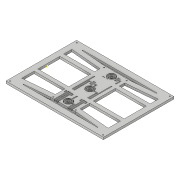
# Autodesk Inventor part: LD_holder_p11
Saved by Autodesk Inventor 2022 (Build 260153000, 153)
## iProperties
Created: 2020-08-30
Part Number: LD_holder_p11
Material: Generic
Document SubType Name: Modeling
Designer: LIU
Density: 1 g/cm^3
Appearance: Default
Author: LIU
Autodesk Inventor part; units mm, degrees
ref_plane "YZ Plane" through (0, 0, 0) normal (1, 0, 0) x (0, 1, 0)
ref_plane "XZ Plane" through (0, 0, 0) normal (0, 1, 0) x (-1, 0, 0)
ref_plane "XY Plane" through (0, 0, 0) normal (0, 0, 1) x (1, 0, 0)
sketch "Sketch1" plane through (0, 0, 0) normal (0, 1, 0) x (-1, 0, 0)
  line L0 (0, -89.88) -> (0, 89.88) construction
  line L1 (124.04, 0) -> (-124.04, 0) construction
  line L2 (0, 15.386221) -> (0, -13.818145) construction
  circle A0 centre (0, 0) radius 1.85
  circle A1 centre (0, -39.2) radius 1.85
  circle A2 centre (0, 39.2) radius 1.85
  line L3 (-22.5, 49.2) -> (22.5, 49.2)
  line L4 (22.5, 49.2) -> (22.5, 40.666307) construction
  line L5 (22.5, -49.2) -> (-22.5, -49.2)
  line L6 (-22.5, -49.2) -> (-22.5, -40.666307) construction
  line L7 (-22.5, 49.2) -> (22.5, -49.2) construction
  line L8 (22.5, 49.2) -> (-22.5, -49.2) construction
  line L9 (-78.6, 54.2) -> (78.6, 54.2)
  line L10 (78.6, 54.2) -> (78.6, 45.666307) construction
  line L11 (78.6, -54.2) -> (-78.6, -54.2)
  line L12 (-78.6, -54.2) -> (-78.6, -45.666307) construction
  line L13 (-78.6, 54.2) -> (78.6, -54.2) construction
  line L14 (78.6, 54.2) -> (-78.6, -54.2) construction
  line L15 (-88.6, 64.2) -> (88.6, 64.2)
  line L16 (88.6, 64.2) -> (88.6, -64.2)
  line L17 (88.6, -64.2) -> (-88.6, -64.2)
  line L18 (-88.6, -64.2) -> (-88.6, 64.2)
  line L19 (-88.6, 64.2) -> (88.6, -64.2) construction
  line L20 (88.6, 64.2) -> (-88.6, -64.2) construction
  line L21 (22.5, -49.2) -> (78.6, -54.2)
  line L22 (22.5, -40.666307) -> (78.6, -45.666307)
  line L23 (22.5, 49.2) -> (78.6, 54.2)
  line L24 (22.5, 40.666307) -> (78.6, 45.666307)
  line L25 (-22.5, -49.2) -> (-78.6, -54.2)
  line L26 (-22.5, -40.666307) -> (-78.6, -45.666307)
  line L27 (-22.5, 40.666307) -> (-78.6, 45.666307)
  line L28 (-22.5, 49.2) -> (-78.6, 54.2)
  circle A3 centre (20.5, 46.2) radius 1
  circle A4 centre (20.5, -46.2) radius 1
  circle A5 centre (-20.5, 46.2) radius 1
  circle A6 centre (-20.5, -46.2) radius 1
  line L29 (78.6, 45.666307) -> (78.6, -45.666307)
  line L30 (78.6, -45.666307) -> (78.6, -54.2) construction
  line L31 (22.5, 40.666307) -> (22.5, -40.666307)
  line L32 (22.5, -40.666307) -> (22.5, -49.2) construction
  line L33 (-22.5, 40.666307) -> (-22.5, 49.2) construction
  line L34 (-22.5, -40.666307) -> (-22.5, 40.666307)
  line L35 (-78.6, 45.666307) -> (-78.6, 54.2) construction
  line L36 (-78.6, -45.666307) -> (-78.6, 45.666307)
  dimension "d0" = 0
  dimension "d1" = 3.7
  dimension "d2" = 3.7
  dimension "d3" = 3.7
  dimension "d4" = 39.2
  dimension "d5" = 39.2
  dimension "d6" = 45
  dimension "d7" = 98.4
  dimension "d8" = 5
  dimension "d9" = 56.1
  dimension "d10" = 10
  dimension "d11" = 10
  dimension "d12" = 8.5
  dimension "d13" = 2
  dimension "d14" = 2
  dimension "d15" = 3
  constraints: 70 end point, 23 parallel, 9 symmetric about line, 7 centre point, 7 midpoint, 7 perpendicular, 5 point on line, 3 horizontal, 1 collinear, 3 other
  measures "d0" distance between parallel lines of L0 L2
  measures "d1" diameter of A0
  measures "d2" diameter of A1
  measures "d3" diameter of A2
  measures "d4" distance of A0.centre A1.centre
  measures "d5" distance of A0.centre A2.centre
  measures "d6" distance of L5.start L5.end
  measures "d7" distance of L3.end L5.start
  measures "d8" distance between parallel lines of L11 L5
  measures "d9" distance between parallel lines of L4 L10
  measures "d10" distance between parallel lines of L16 L10
  measures "d11" distance between parallel lines of L11 L17
  measures "d12" distance between parallel lines of L21 L22
  measures "d13" distance from line of L4 A3.centre
  measures "d14" diameter of A3
  measures "d15" distance from line of L3 A3.centre
extrude "Extrusion1" add sketch "Sketch1" along normal blind 4
fillet "Fillet1" radius 0.5 4 edges at (78.6, 2, 54.2) (-78.6, 2, 54.2) (-78.6, 2, -54.2) (78.6, 2, -54.2)
sketch "Sketch2" plane through (0, 4, 0) normal (0, 1, 0) x (1, 0, 0)
  circle A0 centre (0, -39.2) radius 1.85 projected
  circle A1 centre (0, 39.2) radius 1.85 projected
  circle A2 centre (0, 0) radius 1.85 projected
  circle A3 centre (0, -39.2) radius 2.9
  circle A4 centre (0, 0) radius 2.9
  circle A5 centre (0, 39.2) radius 2.9
  dimension "d19" = 5.8
  dimension "d20" = 5.8
  dimension "d21" = 5.8
  constraints: 3 centre point, 3 coincident
  measures "d19" diameter of A3
  measures "d20" diameter of A4
  measures "d21" diameter of A5
extrude "Extrusion2" cut sketch "Sketch2" against normal blind 1.6
sketch "Sketch3" plane through (0, 4, 0) normal (0, 1, 0) x (1, 0, 0)
  line L0 (-88.6, -64.2) -> (88.6, -64.2) projected
  line L1 (-88.6, 64.2) -> (-88.6, -64.2) projected
  circle A0 centre (-84.6, -60.7) radius 1
  line L2 (0, 89.88) -> (0, -89.88) projected
  line L3 (-124.04, 0) -> (124.04, 0) projected
  circle A1 centre (-84.6, 60.7) radius 1
  circle A2 centre (84.6, -60.7) radius 1
  circle A3 centre (84.6, 60.7) radius 1
  point P0 (0, 0)
  dimension "d24" = 4
  dimension "d25" = 3.5
  dimension "d26" = 2
  constraints: 4 centre point, 3 symmetric about line, 3 other
  measures "d24" distance from line of L1 A0.centre
  measures "d25" distance from line of L0 A0.centre
  measures "d26" diameter of A0
extrude "Extrusion3" cut sketch "Sketch3" against normal through all contours A0 | A1 | A2 | A3
sketch "Sketch4" plane through (0, 0, 0) normal (0, -1, 0) x (1, 0, 0)
  circle A0 centre (84.6, 60.7) radius 1
  circle A1 centre (-84.6, 60.7) radius 1
  circle A2 centre (-84.6, -60.7) radius 1
  circle A3 centre (84.6, -60.7) radius 1
  line L0 (-88.6, 64.2) -> (-88.6, -64.2)
  line L1 (-84.6, -58.332864) -> (-82.55, -59.516432)
  line L2 (-82.55, -59.516432) -> (-82.55, -61.883568)
  line L3 (-82.55, -61.883568) -> (-84.6, -63.067136)
  line L4 (-84.6, -63.067136) -> (-86.65, -61.883568)
  line L5 (-86.65, -61.883568) -> (-86.65, -59.516432)
  line L6 (-86.65, -59.516432) -> (-84.6, -58.332864)
  line L7 (0, -89.88) -> (0, 89.88)
  line L8 (-124.04, 0) -> (124.04, 0)
  circle A4 centre (-84.6, 60.7) radius 1
  line L9 (-84.6, 58.332864) -> (-82.55, 59.516432)
  line L10 (-82.55, 59.516432) -> (-82.55, 61.883568)
  line L11 (-82.55, 61.883568) -> (-84.6, 63.067136)
  line L12 (-84.6, 63.067136) -> (-86.65, 61.883568)
  line L13 (-86.65, 61.883568) -> (-86.65, 59.516432)
  line L14 (-86.65, 59.516432) -> (-84.6, 58.332864)
  circle A5 centre (84.6, 60.7) radius 1
  circle A6 centre (84.6, -60.7) radius 1
  line L15 (84.6, -58.332864) -> (82.55, -59.516432)
  line L16 (82.55, -59.516432) -> (82.55, -61.883568)
  line L17 (82.55, -61.883568) -> (84.6, -63.067136)
  line L18 (84.6, -63.067136) -> (86.65, -61.883568)
  line L19 (86.65, -61.883568) -> (86.65, -59.516432)
  line L20 (86.65, -59.516432) -> (84.6, -58.332864)
  line L21 (84.6, 58.332864) -> (82.55, 59.516432)
  line L22 (86.65, 59.516432) -> (84.6, 58.332864)
  line L23 (82.55, 61.883568) -> (84.6, 63.067136)
  line L24 (86.65, 61.883568) -> (86.65, 59.516432)
  line L25 (82.55, 59.516432) -> (82.55, 61.883568)
  line L26 (84.6, 63.067136) -> (86.65, 61.883568)
  circle A7 centre (84.6, 60.7) radius 1
  point P0 (0, 0)
  dimension "d29" = 4.1
  constraints: 48 end point, 25 symmetric about line, 4 centre point, 4 coincident, 1 parallel, 17 other
  measures "d29" distance between parallel lines of L2 L5
extrude "Extrusion4" cut sketch "Sketch4" against normal blind 2.5
sketch "Sketch6" plane through (0, 4, 0) normal (0, 1, 0) x (1, 0, 0)
  circle A0 centre (0, -39.2) radius 2.9
  line L0 (0, 89.88) -> (0, -89.88)
  line L1 (-124.04, 0) -> (124.04, 0)
  circle A1 centre (0, -39.2) radius 4
  circle A2 centre (0, -39.2) radius 5
  arc A3 (2.296101, -33.656723) -> (0, -33.2) centre (0, -39.2) ccw construction
  arc A4 (2.678784, -32.732843) -> (0, -32.2) centre (0, -39.2) ccw construction
  line L2 (0, -39.2) -> (-2.296101, -33.656723) construction
  line L3 (0, -39.2) -> (2.296101, -33.656723) construction
  line L4 (-2.678784, -32.732843) -> (-5.523371, -25.865402) construction
  arc A5 (0, -45.2) -> (2.296101, -33.656723) centre (0, -39.2) ccw
  arc A6 (0, -46.2) -> (2.678784, -32.732843) centre (0, -39.2) ccw
  arc A7 (-2.296101, -33.656723) -> (0, -45.2) centre (0, -39.2) ccw
  arc A8 (-2.678784, -32.732843) -> (0, -46.2) centre (0, -39.2) ccw
  arc A9 (0, -32.2) -> (-2.678784, -32.732843) centre (0, -39.2) ccw construction
  arc A10 (0, -33.2) -> (-2.296101, -33.656723) centre (0, -39.2) ccw construction
  line L5 (2.296101, -33.656723) -> (2.678784, -32.732843)
  line L6 (2.678784, -32.732843) -> (5.425766, -26.101041) construction
  line L7 (-2.296101, -33.656723) -> (-2.678784, -32.732843)
  circle A11 centre (0, 0) radius 4
  circle A12 centre (0, 0) radius 5
  arc A13 (0, -6) -> (2.296101, 5.543277) centre (0, 0) ccw
  arc A14 (-2.296101, 5.543277) -> (0, -6) centre (0, 0) ccw
  arc A15 (-2.678784, 6.467157) -> (0, -7) centre (0, 0) ccw
  arc A16 (0, -7) -> (2.678784, 6.467157) centre (0, 0) ccw
  line L8 (2.296101, 5.543277) -> (2.678784, 6.467157)
  line L9 (-2.296101, 5.543277) -> (-2.678784, 6.467157)
  circle A17 centre (0, 39.2) radius 4
  circle A18 centre (0, 39.2) radius 5
  arc A19 (2.296101, 33.656723) -> (0, 45.2) centre (0, 39.2) ccw
  arc A20 (2.678784, 32.732843) -> (0, 46.2) centre (0, 39.2) ccw
  arc A21 (0, 45.2) -> (-2.296101, 33.656723) centre (0, 39.2) ccw
  arc A22 (0, 46.2) -> (-2.678784, 32.732843) centre (0, 39.2) ccw
  line L10 (2.296101, 33.656723) -> (2.678784, 32.732843)
  line L11 (-2.296101, 33.656723) -> (-2.678784, 32.732843)
  dimension "d64" = 8
  dimension "d65" = 10
  dimension "d68" = 22.5
  dimension "d69" = 22.5
  dimension "d70" = 6
  dimension "d71" = 7
  dimension "d74" = 39.2
  constraints: 32 point on circle, 22 centre point, 20 end point, 10 coincident, 10 symmetric about line, 5 point on line, 1 collinear, 1 vertical, 24 other
  measures "d64" diameter of A1
  measures "d65" diameter of A2
  measures "d68" angle of L0 L2
  measures "d69" angle of L0 L3
  measures "d70" radius of A7
  measures "d71" radius of A8
  measures "d74" distance of A1.centre A11.centre
extrude "Extrusion6" cut sketch "Sketch6" against normal blind 2 contours A1 L0 A2 | L0 A2 A1 | A20 L10 A19 L0 | L0 A21 L11 A22 | A13 L1 A16 L0 | L0 A15 L1 A14 | A12 L1 A11 L0 | L0 A11 L1 A12 | A13 L8 A16 L1 | L1 A15 L9 A14 | A12 L0 A11 L1 | L1 A11 L0 A12 | A5 L5 A6 L0 | L0 A8 L7 A7 | A18 L0 A17 | L0 A17 A18
sketch "Sketch7" plane through (0, 4, 0) normal (0, 1, 0) x (1, 0, 0)
  line L0 (-22.5, -49.2) -> (22.5, -49.2)
  circle A0 centre (0, 0) radius 5
  arc A1 (2.296101, 33.656723) -> (-2.296101, 33.656723) centre (0, 39.2) ccw
  arc A2 (2.678784, 32.732843) -> (-2.678784, 32.732843) centre (0, 39.2) ccw
  arc A3 (-2.296101, -33.656723) -> (2.296101, -33.656723) centre (0, -39.2) ccw
  arc A4 (-2.678784, -32.732843) -> (2.678784, -32.732843) centre (0, -39.2) ccw
  arc A5 (-2.296101, 5.543277) -> (2.296101, 5.543277) centre (0, 0) ccw
  arc A6 (-2.678784, 6.467157) -> (2.678784, 6.467157) centre (0, 0) ccw
  circle A7 centre (0, -39.2) radius 5
  circle A8 centre (0, 39.2) radius 5
  line L1 (-0.75, -35.1) -> (0.75, -35.1) construction
  line L2 (0.75, -35.1) -> (0.75, -34.25657) construction
  line L3 (0.75, -20.1) -> (-0.75, -20.1)
  line L4 (-0.75, -20.1) -> (-0.75, -21.6) construction
  line L5 (0, 89.88) -> (0, -89.88) construction
  circle A9 centre (0, -39.2) radius 4
  line L6 (-0.75, -34.25657) -> (-0.75, -35.1) construction
  line L7 (0.75, -34.25657) -> (0.75, -20.1)
  line L8 (0.75, -20.1) -> (-10.25, -20.1)
  line L9 (-10.25, -20.1) -> (-10.25, -21.6)
  line L10 (-10.25, -21.6) -> (-8.75, -21.6) construction
  line L11 (0.75, -21.6) -> (0.75, -20.1)
  line L12 (-10.25, -20.1) -> (-8.75, -20.1)
  line L13 (-8.75, -20.1) -> (-8.75, -21.6) construction
  line L14 (-8.75, -49.2) -> (-10.25, -49.2)
  line L15 (-10.25, -49.2) -> (-10.25, -20.1)
  line L16 (-0.75, 4.1) -> (0.75, 4.1) construction
  line L17 (0.75, 4.1) -> (0.75, 4.94343) construction
  line L18 (0.75, 12.1) -> (-0.75, 12.1)
  line L19 (-0.75, 12.1) -> (-0.75, 10.6) construction
  circle A10 centre (0, 0) radius 4
  line L20 (0.75, 12.1) -> (-13.25, 12.1)
  line L21 (-13.25, 12.1) -> (-13.25, 10.6)
  line L22 (-13.25, 10.6) -> (-11.75, 10.6) construction
  line L23 (0.75, 10.6) -> (0.75, 12.1)
  line L24 (-13.25, 12.1) -> (-11.75, 12.1)
  line L25 (-11.75, 12.1) -> (-11.75, 10.6) construction
  line L26 (-11.75, -49.2) -> (-13.25, -49.2)
  line L27 (-13.25, -49.2) -> (-13.25, 12.1)
  circle A11 centre (0, 39.2) radius 4
  line L28 (-0.75, 4.94343) -> (-0.75, 4.1) construction
  line L29 (0.75, 4.94343) -> (0.75, 12.1)
  line L30 (-0.75, -21.6) -> (0.75, -21.6) construction
  line L31 (-0.75, -21.6) -> (-0.75, -34.25657)
  line L32 (-8.75, -21.6) -> (-8.75, -49.2)
  line L33 (-8.75, -21.6) -> (-0.75, -21.6)
  line L34 (-0.75, 10.6) -> (0.75, 10.6) construction
  line L35 (-0.75, 10.6) -> (-0.75, 4.94343)
  line L36 (-11.75, 10.6) -> (-11.75, -49.2)
  line L37 (-11.75, 10.6) -> (-0.75, 10.6)
  line L38 (-0.75, 35.1) -> (0.75, 35.1) construction
  line L39 (0.75, 35.1) -> (0.75, 34.25657) construction
  line L40 (0.75, 27.1) -> (-0.75, 27.1)
  line L41 (-0.75, 27.1) -> (-0.75, 28.6) construction
  line L42 (0.75, 27.1) -> (-14.75, 27.1)
  line L43 (-16.25, 27.1) -> (-16.25, 28.6)
  line L44 (-16.25, 28.6) -> (-0.75, 28.6)
  line L45 (0.75, 28.6) -> (0.75, 27.1)
  line L46 (-16.25, 28.6) -> (-14.75, 28.6)
  line L47 (-14.75, 28.6) -> (-14.75, 27.1) construction
  line L48 (-14.75, -49.2) -> (-16.25, -49.2)
  line L49 (-16.25, -49.2) -> (-16.25, 28.6)
  line L50 (-14.75, 27.1) -> (-14.75, -49.2)
  line L51 (-14.75, 27.1) -> (-16.25, 27.1) construction
  line L52 (-0.75, 28.6) -> (-0.75, 34.25657)
  line L53 (-0.75, 28.6) -> (0.75, 28.6) construction
  line L54 (-0.75, 34.25657) -> (-0.75, 35.1) construction
  line L55 (0.75, 34.25657) -> (0.75, 27.1)
  line L56 (6.1, -39.95) -> (6.959705, -39.95) construction
  line L57 (10.6, -39.95) -> (10.6, -38.45)
  line L58 (10.6, -38.45) -> (6.959705, -38.45)
  line L59 (6.1, -38.45) -> (6.1, -39.95) construction
  line L60 (10.6, -38.45) -> (9.1, -38.45)
  line L61 (9.1, -38.45) -> (9.1, -39.95) construction
  line L62 (9.1, -49.2) -> (10.6, -49.2)
  line L63 (10.6, -49.2) -> (10.6, -38.45)
  line L64 (6.959705, -39.95) -> (9.1, -39.95)
  line L65 (6.959705, -38.45) -> (6.1, -38.45) construction
  line L66 (9.1, -39.95) -> (9.1, -49.2)
  line L67 (9.1, -39.95) -> (10.6, -39.95) construction
  line L68 (6.1, -0.75) -> (6.959705, -0.75) construction
  line L69 (13.6, -0.75) -> (13.6, 0.75)
  line L70 (13.6, 0.75) -> (6.959705, 0.75)
  line L71 (6.1, 0.75) -> (6.1, -0.75) construction
  line L72 (13.6, 0.75) -> (12.1, 0.75)
  line L73 (12.1, 0.75) -> (12.1, -0.75) construction
  line L74 (12.1, -49.2) -> (13.6, -49.2)
  line L75 (13.6, -49.2) -> (13.6, 0.75)
  line L76 (12.1, -0.75) -> (13.6, -0.75) construction
  line L77 (12.1, -0.75) -> (12.1, -49.2)
  line L78 (6.959705, -0.75) -> (12.1, -0.75)
  line L79 (6.959705, 0.75) -> (6.1, 0.75) construction
  line L80 (6.1, 38.45) -> (6.959705, 38.45) construction
  line L81 (16.6, 38.45) -> (16.6, 39.95)
  line L82 (16.6, 39.95) -> (6.959705, 39.95)
  line L83 (6.1, 39.95) -> (6.1, 38.45) construction
  line L84 (16.6, 39.95) -> (15.1, 39.95)
  line L85 (15.1, 39.95) -> (15.1, 38.45) construction
  line L86 (15.1, -49.2) -> (16.6, -49.2)
  line L87 (16.6, -49.2) -> (16.6, 39.95)
  line L88 (15.1, 38.45) -> (15.1, -49.2)
  line L89 (15.1, 38.45) -> (16.6, 38.45) construction
  line L90 (6.959705, 38.45) -> (15.1, 38.45)
  line L91 (6.959705, 39.95) -> (6.1, 39.95) construction
  dimension "d81" = 0.75
  dimension "d82" = 1.5
  dimension "d83" = 0.1
  dimension "d85" = 15
  dimension "d86" = 11
  dimension "d87" = 1.5
  dimension "d88" = 0.1
  dimension "d89" = 1.5
  dimension "d91" = 8
  dimension "d93" = 14
  dimension "d94" = 1.5
  dimension "d95" = 1.5
  dimension "d96" = 1.5
  dimension "d97" = 0.75
  dimension "d98" = 0.1
  dimension "d99" = 0.75
  dimension "d100" = 1.5
  dimension "d101" = 8
  dimension "d102" = 17
  dimension "d103" = 1.5
  dimension "d105" = 1.5
  dimension "d106" = 0.1
  dimension "d107" = 0.75
  dimension "d108" = 1.5
  dimension "d109" = 4.5
  dimension "d110" = 1.5
  dimension "d111" = 0.1
  dimension "d112" = 0.75
  dimension "d113" = 1.5
  dimension "d114" = 7.5
  dimension "d115" = 1.5
  dimension "d116" = 0.1
  dimension "d117" = 0.75
  dimension "d118" = 1.5
  dimension "d119" = 10.5
  dimension "d120" = 1.5
  constraints: 180 end point, 73 parallel, 31 perpendicular, 22 horizontal, 12 point on circle, 6 point on line
  measures "d81" distance between parallel lines of L5 L4
  measures "d82" distance between parallel lines of L4 L2
  measures "d83" distance edge to line of A9 L1
  measures "d85" distance between parallel lines of L1 L3
  measures "d86" distance between parallel lines of L11 L9
  measures "d87" distance between parallel lines of L13 L15
  measures "d88" distance edge to line of A10 L16
  measures "d89" distance between parallel lines of L17 L19
  measures "d91" distance between parallel lines of L16 L18
  measures "d93" distance between parallel lines of L23 L21
  measures "d94" distance between parallel lines of L25 L27
  measures "d95" distance between parallel lines of L8 L10
  measures "d96" distance between parallel lines of L20 L22
  measures "d97" distance between parallel lines of L5 L35
  measures "d98" distance edge to line of A11 L38
  measures "d99" distance between parallel lines of L5 L41
  measures "d100" distance between parallel lines of L41 L39
  measures "d101" distance between parallel lines of L40 L38
  measures "d102" distance of L43.end L45.start
  measures "d103" distance between parallel lines of L42 L44
  measures "d105" distance between parallel lines of L49 L50
  measures "d106" distance edge to line of A3 L59
  measures "d107" distance from line of A4.centre L56
  measures "d108" distance between parallel lines of L58 L56
  measures "d109" distance between parallel lines of L59 L57
  measures "d110" distance between parallel lines of L63 L61
  measures "d111" distance edge to line of A5 L71
  measures "d112" distance from line of L68 A10.centre
  measures "d113" distance between parallel lines of L70 L68
  measures "d114" distance between parallel lines of L69 L71
  measures "d115" distance between parallel lines of L75 L73
  measures "d116" distance edge to line of A1 L83
  measures "d117" distance from line of L80 A11.centre
  measures "d118" distance between parallel lines of L80 L82
  measures "d119" distance between parallel lines of L83 L81
  measures "d120" distance between parallel lines of L87 L85
extrude "Extrusion7" cut sketch "Sketch7" against normal blind 2 contours L49 L43 L44 L52 A8 L55 L45 L40 L42 L50 L0 | L27 L21 L20 L18 L23 L29 A0 L35 L37 L36 L0 | L15 L9 L8 L3 L7 A7 L31 L33 L32 L0 | L66 L64 A4 L58 L57 L63 L0 | L77 L78 A6 L70 L69 L75 L0 | L88 L90 A2 L82 L81 L87 L0
sketch "Sketch8" plane through (0, 4, 0) normal (0, 1, 0) x (1, 0, 0)
  arc A0 (2.678784, 32.732843) -> (6.959705, 38.45) centre (0, 39.2) ccw
  line L0 (2.678784, 32.732843) -> (2.296101, 33.656723)
  arc A1 (2.296101, 33.656723) -> (-2.296101, 33.656723) centre (0, 39.2) ccw
  line L1 (-2.296101, 33.656723) -> (-2.678784, 32.732843)
  line L2 (-10.25, -49.2) -> (-10.25, -20.1)
  line L3 (-0.75, -21.6) -> (-8.75, -21.6)
  arc A2 (-2.678784, -32.732843) -> (6.959705, -39.95) centre (0, -39.2) ccw
  line L4 (-2.678784, -32.732843) -> (-2.296101, -33.656723)
  arc A3 (-2.296101, -33.656723) -> (2.296101, -33.656723) centre (0, -39.2) ccw
  line L5 (2.296101, -33.656723) -> (2.678784, -32.732843)
  line L6 (-2.678784, 6.467157) -> (-2.296101, 5.543277)
  arc A4 (-2.296101, 5.543277) -> (2.296101, 5.543277) centre (0, 0) ccw
  line L7 (2.296101, 5.543277) -> (2.678784, 6.467157)
  circle A5 centre (-9.5, -43.6) radius 0.5
  circle A6 centre (-9.5, -33.6) radius 0.5
  circle A7 centre (-12.5, -43.6) radius 0.5
  circle A8 centre (-12.5, -33.6) radius 0.5
  circle A9 centre (-15.5, -43.6) radius 0.5
  circle A10 centre (-15.5, -33.6) radius 0.5
  line L8 (0, 89.88) -> (0, -89.88)
  circle A11 centre (0, -43.7) radius 0.5
  circle A12 centre (-2.942012, -33.403918) radius 0.5
  circle A13 centre (2.942012, -33.403918) radius 0.5
  circle A14 centre (0, -4.5) radius 0.5
  circle A15 centre (-2.942012, 5.796082) radius 0.5
  circle A16 centre (2.942012, 5.796082) radius 0.5
  circle A17 centre (-2.942012, 33.403918) radius 0.5
  circle A18 centre (2.942012, 33.403918) radius 0.5
  circle A19 centre (0, 43.7) radius 0.5
  dimension "d123" = 1
  dimension "d124" = 1
  dimension "d125" = 10
  dimension "d126" = 0.75
  dimension "d127" = 0.75
  dimension "d128" = 12
  dimension "d134" = 3
  dimension "d141" = 6
  dimension "d143" = 1
  dimension "d144" = 4.5
  dimension "d145" = 1
  dimension "d146" = 1
  dimension "d147" = 1
  dimension "d148" = 4.5
  dimension "d149" = 1
  dimension "d150" = 1
  dimension "d151" = 1
  dimension "d152" = 1
  dimension "d153" = 1
  dimension "d154" = 4.5
  constraints: 15 centre point, 12 tangent, 3 point on line, 2 horizontal, 8 other
  measures "d123" diameter of A5
  measures "d124" diameter of A6
  measures "d125" distance of A6.centre A5.centre
  measures "d126" distance from line of L2 A6.centre
  measures "d127" distance from line of L2 A5.centre
  measures "d128" distance from line of L3 A6.centre
  measures "d134" distance of A5.centre A7.centre
  measures "d141" distance of A5.centre A9.centre
  measures "d143" diameter of A11
  measures "d144" distance of A2.centre A11.centre
  measures "d145" diameter of A12
  measures "d146" diameter of A13
  measures "d147" diameter of A14
  measures "d148" distance of A4.centre A14.centre
  measures "d149" diameter of A15
  measures "d150" diameter of A16
  measures "d151" diameter of A17
  measures "d152" diameter of A18
  measures "d153" diameter of A19
  measures "d154" distance of A0.centre A19.centre
sketch "Sketch8 outline for Extrusion8" plane through (0, 4, 0) normal (0, 1, 0) x (1, 0, 0)
  circle A0 centre (-9.5, -43.6) radius 0.5
  circle A1 centre (-9.5, -33.6) radius 0.5
  circle A2 centre (-12.5, -43.6) radius 0.5
  circle A3 centre (-12.5, -33.6) radius 0.5
  circle A4 centre (-15.5, -43.6) radius 0.5
  circle A5 centre (-15.5, -33.6) radius 0.5
  circle A6 centre (0, -43.7) radius 0.5
  circle A7 centre (-2.942012, -33.403918) radius 0.5
  circle A8 centre (2.942012, -33.403918) radius 0.5
  circle A9 centre (0, -4.5) radius 0.5
  circle A10 centre (-2.942012, 5.796082) radius 0.5
  circle A11 centre (2.942012, 5.796082) radius 0.5
  circle A12 centre (-2.942012, 33.403918) radius 0.5
  circle A13 centre (2.942012, 33.403918) radius 0.5
  circle A14 centre (0, 43.7) radius 0.5
extrude "Extrusion8" cut sketch "Sketch8 outline for Extrusion8" against normal through all
sketch "Sketch9" plane through (0, 4, 0) normal (0, 1, 0) x (1, 0, 0)
  line L0 (15.1, -49.2) -> (15.1, 38.45)
  line L1 (15.1, 38.45) -> (6.959705, 38.45)
  line L2 (6.959705, 39.95) -> (16.6, 39.95)
  line L3 (16.6, 39.95) -> (16.6, -49.2)
  line L4 (-16.25, -49.2) -> (-16.25, 28.6)
  line L5 (-16.25, 28.6) -> (-0.75, 28.6)
  line L6 (0.75, 27.1) -> (-14.75, 27.1)
  line L7 (-13.25, 12.1) -> (0.75, 12.1)
  line L8 (-0.75, 10.6) -> (-11.75, 10.6)
  line L9 (-11.75, 10.6) -> (-11.75, -49.2)
  line L10 (-0.75, -21.6) -> (-8.75, -21.6)
  line L11 (-8.75, -21.6) -> (-8.75, -49.2)
  line L12 (12.1, -49.2) -> (12.1, -0.75)
  line L13 (-7.25, -24.1) -> (-5.75, -24.1)
  line L14 (-5.75, -24.1) -> (-5.75, -28.1)
  line L15 (-5.75, -28.1) -> (-7.25, -28.1)
  line L16 (-7.25, -28.1) -> (-7.25, -24.1)
  line L17 (-19.25, -28.1) -> (-17.75, -28.1)
  line L18 (-17.75, -28.1) -> (-17.75, -24.1)
  line L19 (-17.75, -24.1) -> (-19.25, -24.1)
  line L20 (-19.25, -24.1) -> (-19.25, -28.1)
  line L21 (-8.25, 7.6) -> (-4.25, 7.6)
  line L22 (-4.25, 7.6) -> (-4.25, 9.1)
  line L23 (-4.25, 9.1) -> (-8.25, 9.1)
  line L24 (-8.25, 9.1) -> (-8.25, 7.6)
  line L25 (-8.25, 13.6) -> (-4.25, 13.6)
  line L26 (-4.25, 13.6) -> (-4.25, 15.1)
  line L27 (-4.25, 15.1) -> (-8.25, 15.1)
  line L28 (-8.25, 15.1) -> (-8.25, 13.6)
  line L29 (-8.25, 24.1) -> (-4.25, 24.1)
  line L30 (-4.25, 24.1) -> (-4.25, 25.6)
  line L31 (-4.25, 25.6) -> (-8.25, 25.6)
  line L32 (-8.25, 25.6) -> (-8.25, 24.1)
  line L33 (-8.25, 30.1) -> (-4.25, 30.1)
  line L34 (-4.25, 30.1) -> (-4.25, 31.6)
  line L35 (-4.25, 31.6) -> (-8.25, 31.6)
  line L36 (-8.25, 31.6) -> (-8.25, 30.1)
  line L37 (9.1, -28.1) -> (10.6, -28.1)
  line L38 (10.6, -28.1) -> (10.6, -24.1)
  line L39 (10.6, -24.1) -> (9.1, -24.1)
  line L40 (9.1, -24.1) -> (9.1, -28.1)
  line L41 (18.1, -28.1) -> (19.6, -28.1)
  line L42 (19.6, -28.1) -> (19.6, -24.1)
  line L43 (19.6, -24.1) -> (18.1, -24.1)
  line L44 (18.1, -24.1) -> (18.1, -28.1)
  line L45 (8.6, 35.45) -> (12.6, 35.45)
  line L46 (12.6, 35.45) -> (12.6, 36.95)
  line L47 (12.6, 36.95) -> (8.6, 36.95)
  line L48 (8.6, 36.95) -> (8.6, 35.45)
  line L49 (8.6, 41.45) -> (12.6, 41.45)
  line L50 (12.6, 41.45) -> (12.6, 42.95)
  line L51 (12.6, 42.95) -> (8.6, 42.95)
  line L52 (8.6, 42.95) -> (8.6, 41.45)
  dimension "d157" = 4
  dimension "d158" = 1.5
  dimension "d159" = 2.5
  dimension "d160" = 1.5
  dimension "d161" = 1.5
  dimension "d162" = 1.5
  dimension "d163" = 2.5
  dimension "d164" = 4
  dimension "d165" = 4
  dimension "d166" = 1.5
  dimension "d167" = 1.5
  dimension "d168" = 1.5
  dimension "d169" = 1.5
  dimension "d170" = 3.5
  dimension "d171" = 1.5
  dimension "d172" = 1.5
  dimension "d173" = 1.5
  dimension "d174" = 1.5
  dimension "d175" = 1.5
  dimension "d176" = 4
  dimension "d177" = 1.5
  dimension "d178" = 1.5
  dimension "d179" = 1.5
  dimension "d180" = 2.5
  dimension "d181" = 1.5
  dimension "d182" = 1.5
  dimension "d183" = 4
  dimension "d184" = 1.5
  dimension "d185" = 2.5
  dimension "d186" = 1.5
  constraints: 80 end point, 20 parallel, 10 horizontal, 10 perpendicular, 10 point on line
  measures "d157" distance of L13.end L14.end
  measures "d158" distance between parallel lines of L14 L16
  measures "d159" distance between parallel lines of L13 L10
  measures "d160" distance between parallel lines of L11 L16
  measures "d161" distance between parallel lines of L18 L20
  measures "d162" distance between parallel lines of L4 L18
  measures "d163" distance between parallel lines of L10 L19
  measures "d164" distance between parallel lines of L19 L17
  measures "d165" distance of L21.start L21.end
  measures "d166" distance of L23.end L21.start
  measures "d167" distance between parallel lines of L23 L8
  measures "d168" distance between parallel lines of L7 L25
  measures "d169" distance between parallel lines of L25 L27
  measures "d170" distance between parallel lines of L9 L24
  measures "d171" distance between parallel lines of L31 L6
  measures "d172" distance between parallel lines of L29 L31
  measures "d173" distance between parallel lines of L5 L33
  measures "d174" distance between parallel lines of L33 L35
  measures "d175" distance between parallel lines of L38 L40
  measures "d176" distance of L37.end L38.end
  measures "d177" distance between parallel lines of L12 L38
  measures "d178" distance between parallel lines of L44 L3
  measures "d179" distance between parallel lines of L44 L42
  measures "d180" distance between parallel lines of L39 L10
  measures "d181" distance between parallel lines of L47 L1
  measures "d182" distance of L45.end L46.end
  measures "d183" distance of L45.start L45.end
  measures "d184" distance between parallel lines of L2 L49
  measures "d185" distance between parallel lines of L0 L46
  measures "d186" distance between parallel lines of L49 L51
extrude "Extrusion9" cut sketch "Sketch9" against normal through all
sketch "Sketch10" plane through (-78.6, 0, -45.666307) normal (1, 0, 0) x (0, 0, -1)
  point P0 (-45.666307, 0)
sketch "Sketch11" plane through (88.6, 0, 64.2) normal (1, 0, 0) x (0, 0, -1)
  line L0 (104.866307, 0) -> (23.533693, 0)
  line L1 (41.05368, 0) -> (41.05368, 4)
  line L2 (29.94343, 4) -> (42.6, 4)
  line L3 (64.95, 4) -> (15, 4)
  line L4 (47.822099, 4) -> (47.822099, 0)
  line L5 (47.822099, 0) -> (41.05368, 0)
  line L6 (91.3, 4) -> (15, 4)
  line L7 (87.931245, 4) -> (95.033906, 4)
  line L8 (95.033906, 4) -> (95.033906, 0)
  line L9 (95.033906, 0) -> (87.931245, 0)
  line L10 (87.931245, 0) -> (87.931245, 4)
  point P0 (64.2, 0)
  constraints: 14 end point, 6 point on line, 3 perpendicular, 2 vertical, 1 horizontal
extrude "Extrusion10" add sketch "Sketch11" against normal up to surface (167.2 mm away) contours L0 L10 L6 L7 L8 | L0 L1 L2 L3 L4
body "Solid1"
